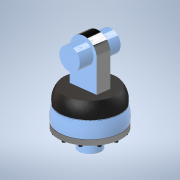
# Autodesk Inventor part: Part6
Saved by Autodesk Inventor 2022 (Build 260153000, 153)
## iProperties
Created: 2023-11-30
Part Number: Part6
Material: Generic
Document SubType Name: Modeling
Designer: harshidd
Density: 1 g/cm^3
Appearance: Red
Author: harshidd
Autodesk Inventor part; units mm, degrees
ref_plane "YZ Plane" through (0, 0, 0) normal (1, 0, 0) x (0, 1, 0)
ref_plane "XZ Plane" through (0, 0, 0) normal (0, 1, 0) x (-1, 0, 0)
ref_plane "XY Plane" through (0, 0, 0) normal (0, 0, 1) x (1, 0, 0)
sketch "Sketch1" plane through (0, 0, 0) normal (0, 0, 1) x (1, 0, 0)
  line L0 (0, 0) -> (-35, 0)
  line L1 (0, 0) -> (0, -20)
  line L2 (0, -20) -> (-40, -20)
  arc A0 (-35, 0) -> (-40, -20) centre (-15.404, -15.524) ccw
  dimension "d0" = 35
  dimension "d1" = 20
  dimension "d2" = 40
  dimension "d3" = 25
  constraints: 6 end point, 2 horizontal, 2 point on circle, 1 centre point, 1 vertical
  measures "d0" distance of L0.start L0.end
  measures "d1" distance of L0.start L1.end
  measures "d2" distance of L1.end L2.end
  measures "d3" radius of A0
revolve "Revolution1" add sketch "Sketch1" angle 360 about axis through (0, 0, 0) along (0, -1, 0)
sketch "Sketch2" plane through (0, -20, 0) normal (0, -1, 0) x (1, 0, 0)
  circle A0 centre (0, 0) radius 39.5
  dimension "d5" = 79
  constraints: 1 centre point, 1 coincident
  measures "d5" diameter of A0
extrude "Extrusion1" add sketch "Sketch2" along normal blind 1
sketch "Sketch3" plane through (0, 0, 0) normal (1, 0, 0) x (0, 1, 0)
  line L0 (-21, 39.5) -> (-21, -39.5) projected
  line L1 (-21, 0) -> (-21, 40)
  line L2 (-21, 0) -> (-41, 0)
  line L3 (-41, 0) -> (-41, 42)
  arc A0 (-21, 40) -> (-41, 42) centre (-34.5432, 5.5677) ccw
  point P0 (0, 0)
  dimension "d8" = 40
  dimension "d9" = 20
  dimension "d10" = 42
  dimension "d11" = 37
  constraints: 6 end point, 2 point on circle, 1 centre point, 1 collinear, 1 horizontal, 1 midpoint, 1 perpendicular
  measures "d8" distance of L1.start L1.end
  measures "d9" distance of L1.start L2.end
  measures "d10" distance of L2.end L3.end
  measures "d11" radius of A0
revolve "Revolution2" add sketch "Sketch3" angle 360 about axis through (0, -21, 0) along (0, -1, 0)
sketch "Sketch4" plane through (0, -41, 0) normal (0, -1, 0) x (1, 0, 0)
  circle A0 centre (0, 0) radius 41.25
  dimension "d13" = 82.5
  constraints: 1 centre point, 1 coincident
  measures "d13" diameter of A0
extrude "Extrusion2" add sketch "Sketch4" along normal blind 0.7
sketch "Sketch5" plane through (0, -41.7, 0) normal (0, -1, 0) x (1, 0, 0)
  circle A0 centre (0, 0) radius 42
  dimension "d16" = 84
  constraints: 1 centre point, 1 coincident
  measures "d16" diameter of A0
extrude "Extrusion3" add sketch "Sketch5" along normal blind 7
sketch "Sketch6" plane through (0, -48.7, 0) normal (0, -1, 0) x (1, 0, 0)
  circle A0 centre (0, 0) radius 35
  dimension "d19" = 70
  constraints: 1 centre point, 1 coincident
  measures "d19" diameter of A0
extrude "Extrusion4" add sketch "Sketch6" along normal blind 3
sketch "Sketch7" plane through (0, -48.7, 0) normal (0, -1, 0) x (1, 0, 0)
  circle A0 centre (0, 0) radius 35 construction
  line L0 (0, -35) -> (0, -42) construction
  circle A1 centre (0, 0) radius 42 construction
  circle A2 centre (0, -38.5) radius 2.25
  dimension "d22" = 4.5
  constraints: 2 end point, 2 vertical alignment, 1 centre point, 1 midpoint, 1 vertical, 2 other
  measures "d22" diameter of A2
extrude "Extrusion5" add sketch "Sketch7" along normal blind 2.7
sketch "Sketch8" plane through (0, -51.4, -38.5) normal (0, -1, 0) x (1, 0, 0)
  circle A0 centre (0, 0) radius 2.25 projected
  circle A1 centre (0, 0) radius 1.55
  point P0 (0, 38.5)
  dimension "d25" = 0.7
  constraints: 1 centre point
  measures "d25" radial gap between concentric circles of A0 A1
extrude "Extrusion6" cut sketch "Sketch8" against normal blind 0.5 contours A1
pattern_circular "Circular Pattern1" count 12 over 360 about axis through (0, -48.7, 0) along (0, -1, 0) of "Extrusion5", "Extrusion6"
sketch "Sketch9" plane through (0, 0, 0) normal (0, 1, 0) x (1, 0, 0)
  line L0 (-10, -20) -> (10, -20)
  line L1 (10, -20) -> (10, 20)
  line L2 (10, 20) -> (-10, 20)
  line L3 (-10, 20) -> (-10, -20)
  line L4 (-10, -20) -> (10, 20) construction
  line L5 (10, -20) -> (-10, 20) construction
  point P0 (0, 0)
  dimension "d31" = 20
  dimension "d32" = 40
  constraints: 12 end point, 2 equal length, 2 midpoint, 1 horizontal, 1 parallel
  measures "d31" distance of L2.end L1.end
  measures "d32" distance of L1.end L0.end
extrude "Extrusion7" add sketch "Sketch9" along normal blind 42
sketch "Sketch10" plane through (10, 0, 20) normal (1, 0, 0) x (0, 0, -1)
  line L0 (0, 42) -> (40, 42) projected
  circle A0 centre (20, 42) radius 20
  point P0 (20, 0)
  constraints: 1 horizontal alignment, 1 midpoint, 2 other
extrude "Extrusion8" add sketch "Sketch10" against normal up to surface (20 mm away)
sketch "Sketch11" plane through (-10, 0, -20) normal (-1, 0, 0) x (0, 0, 1)
  arc A0 (40, 42) -> (0, 42) centre (20, 42) ccw projected
  circle A1 centre (20, 42) radius 15
  point P0 (20, 0)
  dimension "d37" = 30
  constraints: 1 centre point, 1 coincident
  measures "d37" diameter of A1
extrude "Extrusion9" add sketch "Sketch11" along normal blind 20
mirror "Mirror1" about plane through (0, 0, 0) normal (1, 0, 0) of "Extrusion9"
sketch "Sketch12" plane through (0, -51.7, 0) normal (0, -1, 0) x (1, 0, 0)
  circle A0 centre (0, 0) radius 15
  dimension "d40" = 30
  constraints: 1 centre point, 1 coincident
  measures "d40" diameter of A0
extrude "Extrusion10" add sketch "Sketch12" along normal blind 20
body "Solid1"
